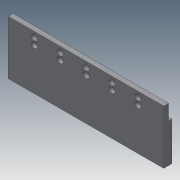
# Autodesk Inventor part: foot bracket foot backside
Saved by Autodesk Inventor 2019 (Build 230136000, 136)
## iProperties
Created: 2019-02-27
Part Number: foot bracket foot backside
Material: Generic
Document SubType Name: Modeling
Designer: LillaHunden
Density: 1 g/cm^3
Appearance: Default
Author: LillaHunden
Autodesk Inventor part; units mm, degrees
ref_plane "YZ Plane" through (0, 0, 0) normal (1, 0, 0) x (0, 1, 0)
ref_plane "XZ Plane" through (0, 0, 0) normal (0, 1, 0) x (-1, 0, 0)
ref_plane "XY Plane" through (0, 0, 0) normal (0, 0, 1) x (1, 0, 0)
sketch "Sketch1" plane through (0, 0, 0) normal (0, 0, 1) x (1, 0, 0)
  line L0 (148.5, -9.5) -> (148.5, -6.2) construction
  line L1 (148.5, -6.2) -> (193, -6.2) construction
  line L2 (193, 9.5) -> (193, -6.2) construction
  line L3 (0, 9.5) -> (193, 9.5) construction
  line L4 (0, -9.5) -> (0, 9.5) construction
  line L5 (148.5, -9.5) -> (0, -9.5) construction
  line L6 (0, 9.5) -> (193, 9.5)
  line L7 (193, 9.5) -> (193, -57.5)
  line L8 (193, -57.5) -> (0, -57.5)
  line L9 (0, -57.5) -> (0, 9.5)
  circle A0 centre (128.6667, -4.8333) radius 1.621 projected
  circle A1 centre (96.5, 3.1667) radius 1.621 projected
  circle A2 centre (64.3333, -4.8333) radius 1.621 projected
  circle A3 centre (32.1667, 3.1667) radius 1.621 projected
  circle A4 centre (32.1667, -4.8333) radius 1.621 projected
  circle A5 centre (64.3333, 3.1667) radius 1.621 projected
  circle A6 centre (96.5, -4.8333) radius 1.621 projected
  circle A7 centre (128.6667, 3.1667) radius 1.621 projected
  circle A8 centre (160.8333, 3.1667) radius 1.621 projected
  point P0 (0, 0)
  constraints: 8 end point, 2 parallel, 1 horizontal, 1 perpendicular
extrude "Extrusion1" add sketch "Sketch1" along normal blind 10 contours L6 L7 L8 L9 | A0 | A1 | A2 | A3 | A4 | A5 | A6 | A7 | A8
sketch "Sketch2" plane through (0, -57.5, 0) normal (-1, 0, 0) x (0, 0, 1)
  line L0 (-111.7541, 55) -> (-111.7541, 67) construction
  line L1 (-116, 67) -> (-111.7541, 67) construction
  line L2 (-116, 48) -> (-116, 67) construction
  line L3 (4, 48) -> (-116, 48) construction
  line L4 (4, 48) -> (4, 67) construction
  line L5 (-54.7541, 67) -> (4, 67) construction
  line L6 (-54.7541, 67) -> (-54.7541, 55) construction
  line L7 (-54.7541, 55) -> (-111.7541, 55) construction
  line L8 (0, 67) -> (0, 0) projected
  line L9 (4, 67) -> (0, 67)
  line L10 (0, 67) -> (0, 48)
  line L11 (0, 48) -> (4, 48)
  line L12 (4, 48) -> (4, 67)
  point P0 (0, 57.5)
  constraints: 8 end point, 2 parallel, 2 point on line, 1 horizontal, 1 perpendicular
extrude "Extrusion2" cut sketch "Sketch2" against normal through all
sketch "Sketch3" plane through (0, 0, 10) normal (0, 0, 1) x (1, 0, 0)
  line L0 (193, -9.5) -> (193, 9.5) projected
  line L1 (0, -9.5) -> (193, -9.5) projected
  line L2 (0, 9.5) -> (0, -9.5) projected
  line L3 (193, 9.5) -> (0, 9.5) projected
  line L4 (0, 0) -> (193, 0) construction
  point P0 (32.1667, 3.1667)
  point P1 (64.3333, 3.1667)
  point P2 (96.5, 3.1667)
  point P3 (128.6667, 3.1667)
  point P4 (160.8333, 3.1667)
  point P5 (32.1667, -4.8333)
  point P6 (64.3333, -4.8333)
  point P7 (96.5, -4.8333)
  point P8 (128.6667, -4.8333)
  point P9 (160.8333, -4.8333)
  dimension "d4" = 32.1667
  dimension "d5" = 32.1667
  dimension "d6" = 32.1667
  dimension "d7" = 32.1667
  dimension "d8" = 32.1667
  dimension "d9" = 8
  dimension "d10" = 6.3333
  constraints: 5 vertical alignment, 4 horizontal alignment, 2 end point, 1 midpoint
  measures "d4" distance of point (64.333, 3.167) point (32.167, 3.167)
  measures "d5" distance from line of L2 point (32.167, 3.167)
  measures "d6" distance of point (96.5, 3.167) point (64.333, 3.167)
  measures "d7" distance of point (96.5, 3.167) point (128.667, 3.167)
  measures "d8" distance of point (128.667, 3.167) point (160.833, 3.167)
  measures "d9" distance of point (32.167, 3.167) point (32.167, -4.833)
  measures "d10" distance from line of L3 point (32.167, 3.167)
hole "Hole1" at (32.1667, 3.1667, 10) at (64.3333, 3.1667, 10) at (96.5, 3.1667, 10) at (128.6667, 3.1667, 10) at (160.8333, 3.1667, 10) at (32.1667, -4.8333, 10) at (64.3333, -4.8333, 10) at (96.5, -4.8333, 10) at (128.6667, -4.8333, 10) direction (0, 0, -1) diameter 4.5 depth 14.2 counterbore diameter 8 counterbore depth 4.6 clearance for "Socket Head Cap Screw ISO 4762" size "M4" standard "ISO"
equation "\"d5\" = d4"
equation "\"d6\" = d4"
equation "\"d7\" = d6"
equation "\"d8\" = d7"
body "Solid1"
